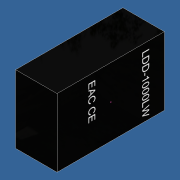
# Autodesk Inventor part: LDD-1000LW
Saved by Autodesk Inventor 2018.2 (Build 222227000, 227)
## iProperties
Created: 2018-10-31
Part Number: LDD-1000LW
Material: Kst - PTFE(white)
Document SubType Name: Modeling
Designer: N.Grubert
Density: 2.16 g/cm^3
Appearance: Plastik (Teflon)
Fläche: 0 cm²
Gewicht: 0 g
Material: geeigneten Werkstoff auswählen !
Dateiname: P:\INVENTOR\Inventor 2018\Templates\ILT\Norm.ipt
Bez_eng: bolt
Bez_french: boulon
Author: N.Grubert
Autodesk Inventor part; units mm, degrees
ref_plane "YZ Plane" through (0, 0, 0) normal (1, 0, 0) x (0, 1, 0)
ref_plane "XZ Plane" through (0, 0, 0) normal (0, 1, 0) x (-1, 0, 0)
ref_plane "XY Plane" through (0, 0, 0) normal (0, 0, 1) x (1, 0, 0)
sketch "Skizze4" plane through (0, 0, 0) normal (1, 0, 0) x (0, 1, 0)
  line L0 (-15.675, 9.95) -> (15.675, 9.95)
  line L1 (15.675, 9.95) -> (15.675, -9.95)
  line L2 (15.675, -9.95) -> (-15.675, -9.95)
  line L3 (-15.675, -9.95) -> (-15.675, 9.95)
  line L4 (0, -13.93) -> (0, 13.93) construction
  line L5 (-21.945, 0) -> (21.945, 0) construction
  point P0 (0, 0)
  dimension "d4" = 31.35
  dimension "d5" = 19.9
  constraints: 8 end point, 2 parallel, 1 horizontal, 1 perpendicular, 2 other
  measures "d4" distance between parallel lines of L1 L3
  measures "d5" distance of L0.end L1.end
extrude "Extrusion2" add sketch "Skizze4" along normal blind 12.1
sketch "Skizze5" plane through (0, 0, 0) normal (0, 1, 0) x (-1, 0, 0)
  circle A0 centre (0, 0) radius 2
  dimension "d8" = 4
  constraints: 1 centre point, 1 coincident
  measures "d8" diameter of A0
extrude "Extrusion3" cut sketch "Skizze5" along normal mid plane 20
fillet "Rundung1" radius 2 2 edges at (2, -10, 0) (2, 10, 0)
sketch "Skizze6" plane through (0, 0, 0) normal (-1, 0, 0) x (0, 0, 1)
  line L0 (-6.95, 7.675) -> (-6.95, -12.325) construction
  line L1 (9.95, 15.675) -> (-9.95, 15.675) construction
  line L2 (-9.95, 15.675) -> (-9.95, -15.675) construction
  line L3 (-6.95, 11.675) -> (6.95, 11.675) construction
  line L4 (6.95, 11.675) -> (6.95, -12.325) construction
  line L5 (9.95, -15.675) -> (9.95, 15.675) construction
  point P0 (0, 0)
  dimension "d12" = 4
  dimension "d15" = 4
  dimension "d16" = 24
  dimension "d17" = 3
  dimension "d18" = 24
  dimension "d19" = 3
  constraints: 6 end point, 3 perpendicular, 1 horizontal, 1 point on line, 1 vertical
  measures "d12" distance of L0.start L3.start
  measures "d15" distance from line of L1 L3.start
  measures "d16" distance of L0.end L3.start
  measures "d17" distance from line of L2 L3.start
  measures "d18" distance of L4.end L3.end
  measures "d19" distance from line of L5 L3.end
hole "Bohrung1" at (0, 7.675, -6.95) at (0, 11.675, -6.95) at (0, -12.325, -6.95) at (0, 11.675, 6.95) at (0, -12.325, 6.95) direction (1, 0, 0) diameter 1 depth 2 tip angle 118
sketch "Skizze7" plane through (12.1, 0, 0) normal (1, 0, 0) x (0, 0, -1)
  line L0 (-8.0362, 11.2286) -> (8.4274, 11.2286) construction
  line L1 (8.4274, 11.2286) -> (8.4274, -13.5124) construction
  line L2 (8.4274, -13.5124) -> (-8.0362, -13.5124) construction
  line L3 (-8.0362, -13.5124) -> (-8.0362, 11.2286) construction
  point P0 (0, 0)
  constraints: 2 other
equation "\"d19\" = d17"
